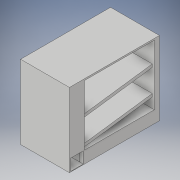
# Autodesk Inventor part: OUTER CASE
Saved by Autodesk Inventor 2019 (Build 230136000, 136)
## iProperties
Created: 2020-03-10
Part Number: OUTER CASE
Material: Generic
Document SubType Name: Modeling
Designer: Hp
Density: 1 g/cm^3
Appearance: Default
Author: Hp
Autodesk Inventor part; units mm, degrees
ref_plane "YZ Plane" through (0, 0, 0) normal (1, 0, 0) x (0, 1, 0)
ref_plane "XZ Plane" through (0, 0, 0) normal (0, 1, 0) x (-1, 0, 0)
ref_plane "XY Plane" through (0, 0, 0) normal (0, 0, 1) x (1, 0, 0)
sketch "Sketch1" plane through (0, 0, 0) normal (1, 0, 0) x (0, 1, 0)
  line L0 (17.9465, 50) -> (-182.0535, 50)
  line L1 (-182.0535, 50) -> (-182.0535, -300)
  line L2 (-182.0535, -300) -> (17.9465, -300)
  line L3 (17.9465, -300) -> (17.9465, 50)
  point P0 (0, 0)
  dimension "d0" = 200
  dimension "d1" = 350
  constraints: 8 end point, 2 parallel, 1 horizontal, 1 perpendicular
  measures "d0" distance of L2.end L1.end
  measures "d1" distance of L1.end L0.end
extrude "Extrusion1" add sketch "Sketch1" along normal blind 5
sketch "Sketch2" plane through (5, 0, 0) normal (1, 0, 0) x (0, 0, -1)
  circle A0 centre (35, -35.893) radius 14
  line L0 (-50, 17.9465) -> (-50, -182.0535) projected
  line L1 (132.0128, -157.8668) -> (156.8147, -157.8668)
  circle A1 centre (80, -35.893) radius 14
  circle A2 centre (125, -35.893) radius 14
  circle A3 centre (170, -35.893) radius 14
  circle A4 centre (215, -35.893) radius 14
  point P0 (0, 0)
  dimension "d4" = 28
  dimension "d5" = 85
  dimension "d8" = 45
  constraints: 5 centre point, 2 end point, 2 horizontal, 9 other
  measures "d4" diameter of A0
  measures "d8" distance of A0.centre A1.centre
extrude "Extrusion2" cut sketch "Sketch2" against normal blind 1
sketch "Sketch4" plane through (5, 0, 0) normal (1, 0, 0) x (0, 0, -1)
  line L0 (-50, 17.9465) -> (-50, -182.0535) projected
  line L1 (-50, -182.0535) -> (300, -182.0535) projected
  line L2 (-50, 17.9465) -> (0, 17.9465)
  line L3 (0, 17.9465) -> (0, -182.0535)
  line L4 (0, -182.0535) -> (-50, -182.0535)
  line L5 (-50, -182.0535) -> (-50, 17.9465)
  point P0 (0, 0)
  dimension "d17" = 50
  constraints: 8 end point, 2 parallel, 1 horizontal, 1 perpendicular, 1 point on line, 1 other
extrude "Extrusion3" add sketch "Sketch4" along normal blind 150
sketch "Sketch5" plane through (5, 0, 0) normal (1, 0, 0) x (0, 0, -1)
  circle A0 centre (35, -122.0535) radius 14
  line L0 (0, -182.0535) -> (300, -182.0535) projected
  circle A1 centre (80, -122.0535) radius 14
  circle A2 centre (125, -122.0535) radius 14
  circle A3 centre (170, -122.0535) radius 14
  circle A4 centre (215, -122.0535) radius 14
  point P0 (0, 0)
  dimension "d18" = 28
  dimension "d19" = 60
  dimension "d22" = 45
  constraints: 5 centre point, 1 horizontal, 8 other
  measures "d18" diameter of A0
  measures "d19" distance from line of L0 A0.centre
  measures "d22" distance of A0.centre A1.centre
extrude "Extrusion4" cut sketch "Sketch5" against normal blind 2
sketch "Sketch6" plane through (5, 0, 0) normal (1, 0, 0) x (0, 0, -1)
  line L0 (0, -182.0535) -> (300, -182.0535) projected
  line L1 (299.7409, 17.9465) -> (246.5216, 17.9465)
  line L2 (246.5216, 17.9465) -> (246.5216, -182.0535)
  line L3 (246.5216, -182.0535) -> (299.7409, -182.0535)
  line L4 (299.7409, -182.0535) -> (299.7409, 17.9465)
  point P0 (0, 0)
  dimension "d29" = 200
  constraints: 8 end point, 2 parallel, 1 horizontal, 1 perpendicular, 1 point on line
  measures "d29" distance of L3.end L1.start
extrude "Extrusion5" cut sketch "Sketch6" against normal blind 20
sketch "Sketch7" plane through (5, 0, 0) normal (1, 0, 0) x (0, 0, -1)
  line L0 (290.724, 51.1324) -> (325.2992, 51.1324)
  line L1 (325.2992, 51.1324) -> (325.2992, -191.8681)
  line L2 (325.2992, -191.8681) -> (290.724, -191.8681)
  line L3 (290.724, -191.8681) -> (290.724, 51.1324)
  point P0 (0, 0)
  constraints: 8 end point, 2 parallel, 1 horizontal, 1 perpendicular
extrude "Extrusion6" cut sketch "Sketch7" against normal blind 20
sketch "Sketch8" plane through (5, 0, 0) normal (1, 0, 0) x (0, 0, -1)
  line L0 (0, -182.0535) -> (246.5216, -182.0535) projected
  line L1 (246.8963, 18.505) -> (231.8963, 18.505)
  line L2 (231.8963, 18.505) -> (231.8963, -182.0535)
  line L3 (231.8963, -182.0535) -> (246.8963, -182.0535)
  line L4 (246.8963, -182.0535) -> (246.8963, 18.505)
  point P0 (0, 0)
  dimension "d34" = 15
  constraints: 8 end point, 2 parallel, 1 horizontal, 1 perpendicular, 1 point on line
  measures "d34" distance of L3.end L2.end
extrude "Extrusion7" add sketch "Sketch8" along normal blind 150
sketch "Sketch9" plane through (5, -182.0535, 0) normal (0, 0, -1) x (-1, 0, 0)
  point P0 (5, 182.0535)
sketch "Sketch10" plane through (5, 0, 0) normal (1, 0, 0) x (0, 0, -1)
  line L0 (0, -182.0535) -> (0, 17.9465) projected
  line L1 (0, -85.1802) -> (231.8963, -53.9271)
  line L2 (231.8963, -182.0535) -> (231.8963, 17.9465) projected
  line L3 (231.8963, -53.9271) -> (231.8963, -63.9271)
  line L4 (0, -85.1802) -> (0, -95.1802)
  line L5 (0, -95.1802) -> (231.8963, -63.9271)
  line L6 (0, -170.1802) -> (231.8963, -138.9271)
  line L7 (0, -180.1802) -> (231.8963, -148.9271)
  line L8 (0, -170.1802) -> (0, -180.1802)
  line L9 (231.8963, -138.9271) -> (231.8963, -148.9271)
  point P0 (0, 0)
  dimension "d37" = 10
  dimension "d38" = 10
  dimension "d41" = 85
  constraints: 16 end point, 4 point on line, 1 vertical, 8 other
  measures "d37" distance of L1.end L3.end
  measures "d38" distance of L1.start L4.end
  measures "d41" distance of L1.start L6.start
extrude "Extrusion8" add sketch "Sketch10" along normal blind 150 contours L0 L6 L2 L7 | L0 L1 L2 L5
sketch "Sketch11" plane through (0, -182.0535, 50) normal (0, -1, 0) x (1, 0, 0)
  line L0 (150.9028, -4.3641) -> (4.8678, -4.3641)
  line L1 (4.8678, -4.3641) -> (4.8678, -45.7406)
  line L2 (4.8678, -45.7406) -> (150.9028, -45.7406)
  line L3 (150.9028, -45.7406) -> (150.9028, -4.3641)
  point P0 (0, -50)
  constraints: 8 end point, 2 parallel, 1 horizontal, 1 perpendicular
extrude "Extrusion9" cut sketch "Sketch11" against normal blind 190
sketch "Sketch12" plane through (155, 17.9465, 0) normal (0, 0, -1) x (-1, 0, 0)
  line L0 (150, -103.1268) -> (150, -71.8736) projected
  line L1 (150, -103.1268) -> (0, -103.1268)
  line L2 (0, -103.1268) -> (0, -83.1268)
  line L3 (0, -83.1268) -> (150, -83.1268)
  line L4 (150, -83.1268) -> (150, -103.1268)
  line L5 (0, -103.1268) -> (0, 0) projected
  line L6 (150, -188.1268) -> (0, -188.1268)
  line L7 (0, -188.1268) -> (0, -168.1268)
  line L8 (0, -168.1268) -> (150, -168.1268)
  line L9 (150, -168.1268) -> (150, -188.1268)
  point P0 (155, -17.9465)
  dimension "d50" = 20
  dimension "d51" = 0
  dimension "d54" = 85
  constraints: 16 end point, 2 parallel, 1 collinear, 1 horizontal, 1 perpendicular, 1 vertical, 7 other
  measures "d50" distance between parallel lines of L1 L3
  measures "d51" distance between parallel lines of L5 L2
  measures "d54" distance of L2.end L7.end
extrude "Extrusion10" cut sketch "Sketch12" against normal blind 7
fillet "Fillet1" radius 5 2 edges at (77.9514, -85.1802, 4.2594) (77.9514, -170.1802, 4.2594)
sketch "Sketch13" plane through (0, -182.0535, 50) normal (0, -1, 0) x (1, 0, 0)
  line L0 (0, 0) -> (155, 0) projected
  line L1 (0, -296.5216) -> (0, 0) projected
  line L2 (155, 0) -> (0, 0)
  line L3 (0, 0) -> (0, -296.5216)
  line L4 (0, -296.5216) -> (155, -296.5216)
  line L5 (155, -296.5216) -> (155, 0)
  line L6 (4.8678, -4.3641) -> (150.9028, -4.3641) projected
  line L7 (5, -50) -> (5, -45.7406) projected
  line L8 (150.9028, -4.3641) -> (5, -4.3641)
  line L9 (5, -4.3641) -> (5, -45.7406)
  line L10 (5, -45.7406) -> (150.9028, -45.7406)
  line L11 (150.9028, -45.7406) -> (150.9028, -4.3641)
  point P0 (0, -50)
  constraints: 16 end point, 4 parallel, 2 horizontal, 2 perpendicular
extrude "Extrusion11" add sketch "Sketch13" along normal blind 40
sketch "Sketch14" plane through (0, 17.9465, 50) normal (0, 1, 0) x (1, 0, 0)
  line L0 (0, 296.5216) -> (155, 296.5216) projected
  line L1 (0, 0) -> (155, 0)
  line L2 (155, 0) -> (155, 296.5216)
  line L3 (155, 296.5216) -> (0, 296.5216)
  line L4 (0, 296.5216) -> (0, 0)
  point P0 (0, 50)
  constraints: 8 end point, 2 parallel, 1 horizontal, 1 perpendicular
extrude "Extrusion12" add sketch "Sketch14" along normal blind 5
sketch "Sketch15" plane through (155, 18.505, -246.5216) normal (0, 0, -1) x (-1, 0, 0)
  line L0 (155, -240.5585) -> (0, -240.5585) projected
  line L1 (0, -240.5585) -> (155, -240.5585)
  line L2 (155, -240.5585) -> (155, 4.4415)
  line L3 (155, 4.4415) -> (0, 4.4415)
  line L4 (0, 4.4415) -> (0, -240.5585)
  line L5 (0, 4.4415) -> (155, 4.4415) projected
  point P0 (155, -18.505)
  dimension "d66" = 0
  constraints: 8 end point, 2 parallel, 1 horizontal, 1 perpendicular
  measures "d66" distance between parallel lines of L5 L3
extrude "Extrusion13" add sketch "Sketch15" along normal blind 2
sketch "Sketch16" plane through (155, 0, 0) normal (1, 0, 0) x (0, 0, -1)
  line L0 (-50, -222.0535) -> (-50, 22.9465) projected
  line L1 (-50, -222.0535) -> (248.5216, -222.0535) projected
  line L2 (-50, 22.9465) -> (248.5216, 22.9465)
  line L3 (248.5216, 22.9465) -> (248.5216, -222.0535)
  line L4 (248.5216, -222.0535) -> (-50, -222.0535)
  line L5 (-50, -222.0535) -> (-50, 22.9465)
  line L6 (0, 17.9465) -> (0, -65.1802) projected
  line L7 (231.8963, -182.0535) -> (0, -182.0535) projected
  line L8 (0, 17.9465) -> (231.8963, 17.9465)
  line L9 (231.8963, 17.9465) -> (231.8963, -182.0535)
  line L10 (231.8963, -182.0535) -> (0, -182.0535)
  line L11 (0, -182.0535) -> (0, 17.9465)
  point P0 (0, 0)
  constraints: 16 end point, 4 parallel, 2 horizontal, 2 perpendicular
extrude "Extrusion14" add sketch "Sketch16" along normal blind 7
sketch "Sketch17" plane through (162, 0, 0) normal (1, 0, 0) x (0, 0, -1)
  line L0 (-50, -222.0535) -> (248.5216, -222.0535) projected
  line L1 (-45.6359, -182.0535) -> (-45.6359, 7.9465) projected
  line L2 (-4.5693, -222.0535) -> (-45.6359, -222.0535)
  line L3 (-45.6359, -222.0535) -> (-45.6359, -182.0535)
  line L4 (-45.6359, -182.0535) -> (-4.5693, -182.0535)
  line L5 (-4.5693, -182.0535) -> (-4.5693, -222.0535)
  point P0 (0, 0)
  constraints: 8 end point, 2 parallel, 1 horizontal, 1 perpendicular, 1 point on line
extrude "Extrusion15" cut sketch "Sketch17" against normal blind 50
sketch "Sketch18" plane through (0, -222.0535, 50) normal (0, -1, 0) x (1, 0, 0)
  line L0 (162, -298.5216) -> (162, 0) projected
  line L1 (0, 0) -> (162, 0)
  line L2 (162, 0) -> (162, -298.5216)
  line L3 (162, -298.5216) -> (0, -298.5216)
  line L4 (0, -298.5216) -> (0, 0)
  point P0 (0, -50)
  constraints: 8 end point, 2 parallel, 1 horizontal, 1 perpendicular
extrude "Extrusion16" add sketch "Sketch18" against normal blind 2
body "Solid1"
